Autodesk Fusion 360 part; units mm, degrees
note: some values were not read from the file. Set by a fixed rule: which sketch regions a step uses.
(part 2 of 4)
sketch "Sketch1 (2)" plane through (0, 0, 10) normal (0, 0, 1) x (-1, 0, 0)
  arc A0 (-15.295851, 2.795456) -> (-15.3295, 2.604619) centre (0, 0) ccw
  arc A1 (-16.525343, 1.694532) -> (-15.3295, 2.604619) centre (-16.413958, 2.788878) ccw
  line L0 (-16.525343, 1.694532) -> (-16.82626, 1.72516)
  spline S0 degree 3 poles (-19.988384, 0.681532) (-19.542306, 0.942193) (-19.068507, 1.175344) (-17.814234, 1.647532) (-17.303236, 1.701034) (-16.95637, 1.733314) (-16.879441, 1.730573) (-16.82626, 1.72516) knots -0.0362684 -0.0362684 -0.0362684 -0.0362684 -0.0284651 -0.0284651 -0.01603664 -0.01603664 0 0 0 0
  arc A2 (-19.988384, 0.681532) -> (-19.988384, -0.681532) centre (0, 0) ccw
  spline S1 degree 3 poles (-16.82626, -1.72516) (-17.047028, -1.747631) (-17.379442, -1.693217) (-17.83236, -1.598794) (-18.095918, -1.53109) (-18.963438, -1.226643) (-19.493456, -0.970738) (-19.988384, -0.681532) knots -0.3979886 -0.3979886 -0.3979886 -0.3979886 -0.27573533 -0.27573533 -0.17196952 -0.17196952 0 0 0 0
  line L1 (-16.82626, -1.72516) -> (-16.525343, -1.694532)
  arc A3 (-15.3295, -2.604619) -> (-16.525343, -1.694532) centre (-16.413958, -2.788878) ccw
  arc A4 (-15.3295, -2.604619) -> (-15.295851, -2.795456) centre (0, 0) ccw
  arc A5 (-16.108307, -4.059661) -> (-15.295851, -2.795456) centre (-16.377928, -2.993216) ccw
  line L2 (-16.108307, -4.059661) -> (-16.401552, -4.133799)
  spline S2 degree 3 poles (-19.016035, -6.196) (-18.68601, -5.79849) (-18.320527, -5.417351) (-17.303393, -4.544654) (-16.841511, -4.319606) (-16.526604, -4.170638) (-16.453377, -4.146902) (-16.401552, -4.133799) knots -0.0362684 -0.0362684 -0.0362684 -0.0362684 -0.0284651 -0.0284651 -0.01603664 -0.01603664 0 0 0 0
  arc A6 (-19.016035, -6.196) -> (-18.54984, -7.476861) centre (0, 0) ccw
  spline S3 degree 3 poles (-15.221473, -7.37604) (-15.421242, -7.472663) (-15.752219, -7.535223) (-16.210117, -7.601402) (-16.480937, -7.627923) (-17.400266, -7.638545) (-17.985845, -7.57935) (-18.54984, -7.476861) knots -0.3979886 -0.3979886 -0.3979886 -0.3979886 -0.27573533 -0.27573533 -0.17196952 -0.17196952 0 0 0 0
  line L3 (-15.221473, -7.37604) -> (-14.949179, -7.24434)
  arc A7 (-13.514186, -7.690539) -> (-14.949179, -7.24434) centre (-14.470223, -8.234593) ccw
  arc A8 (-13.514186, -7.690539) -> (-13.417296, -7.858359) centre (0, 0) ccw
  arc A9 (-13.748372, -9.324199) -> (-13.417296, -7.858359) centre (-14.366478, -8.414284) ccw
  line L4 (-13.748372, -9.324199) -> (-13.998575, -9.494162)
  spline S4 degree 3 poles (-15.750071, -12.326202) (-15.575905, -11.83979) (-15.36282, -11.356634) (-14.705508, -10.188687) (-14.348452, -9.819238) (-14.103485, -9.571549) (-14.042793, -9.524199) (-13.998575, -9.494162) knots -0.0362684 -0.0362684 -0.0362684 -0.0362684 -0.0284651 -0.0284651 -0.01603664 -0.01603664 0 0 0 0
  arc A10 (-15.750071, -12.326202) -> (-14.873911, -13.37037) centre (0, 0) ccw
  spline S5 degree 3 poles (-11.780751, -12.137261) (-11.935426, -12.296381) (-12.225046, -12.46837) (-12.632695, -12.687167) (-12.878111, -12.804715) (-13.738365, -13.129126) (-14.308875, -13.27378) (-14.873911, -13.37037) knots -0.3979886 -0.3979886 -0.3979886 -0.3979886 -0.27573533 -0.27573533 -0.17196952 -0.17196952 0 0 0 0
  line L5 (-11.780751, -12.137261) -> (-11.569923, -11.920373)
  arc A11 (-10.068861, -11.848867) -> (-11.569923, -11.920373) centre (-10.781165, -12.687094) ccw
  arc A12 (-10.068861, -11.848867) -> (-9.920417, -11.973427) centre (0, 0) ccw
  arc A13 (-9.73018, -13.464101) -> (-9.920417, -11.973427) centre (-10.622219, -12.820465) ccw
  line L6 (-9.73018, -13.464101) -> (-9.907163, -13.709388)
  spline S6 degree 3 poles (-10.584416, -16.969683) (-10.587116, -16.453037) (-10.552131, -15.92614) (-10.333921, -14.603813) (-10.124757, -14.134525) (-9.979279, -13.81799) (-9.938441, -13.752738) (-9.907163, -13.709388) knots -0.0362684 -0.0362684 -0.0362684 -0.0362684 -0.0284651 -0.0284651 -0.01603664 -0.01603664 0 0 0 0
  arc A14 (-10.584416, -16.969683) -> (-9.403968, -17.651215) centre (0, 0) ccw
  spline S7 degree 3 poles (-6.919097, -15.434549) (-7.010021, -15.636975) (-7.223352, -15.897647) (-7.531583, -16.242674) (-7.721996, -16.43707) (-8.419415, -17.03614) (-8.906044, -17.367197) (-9.403968, -17.651215) knots -0.3979886 -0.3979886 -0.3979886 -0.3979886 -0.27573533 -0.27573533 -0.17196952 -0.17196952 0 0 0 0
  line L7 (-6.919097, -15.434549) -> (-6.795164, -15.158633)
  arc A15 (-5.409084, -14.578046) -> (-6.795164, -15.158633) centre (-5.791739, -15.609344) ccw
  arc A16 (-5.409084, -14.578046) -> (-5.226989, -14.644323) centre (0, 0) ccw
  arc A17 (-4.538384, -15.980034) -> (-5.226989, -14.644323) centre (-5.596763, -15.680309) ccw
  line L8 (-4.538384, -15.980034) -> (-4.620801, -16.27106)
  spline S8 degree 3 poles (-4.142124, -19.566369) (-4.321365, -19.081804) (-4.468699, -18.574717) (-4.715911, -17.257505) (-4.679867, -16.74498) (-4.651423, -16.397778) (-4.635366, -16.322493) (-4.620801, -16.27106) knots -0.0362684 -0.0362684 -0.0362684 -0.0362684 -0.0284651 -0.0284651 -0.01603664 -0.01603664 0 0 0 0
  arc A18 (-4.142124, -19.566369) -> (-2.799769, -19.803063) centre (0, 0) ccw
  spline S9 degree 3 poles (-1.222898, -16.870202) (-1.239105, -17.091518) (-1.350415, -17.409433) (-1.522052, -17.839074) (-1.634494, -18.086871) (-2.084959, -18.888345) (-2.429013, -19.365873) (-2.799769, -19.803063) knots -0.3979886 -0.3979886 -0.3979886 -0.3979886 -0.27573533 -0.27573533 -0.17196952 -0.17196952 0 0 0 0
  line L9 (-1.222898, -16.870202) -> (-1.200807, -16.568538)
  arc A19 (-0.09689, -15.548898) -> (-1.200807, -16.568538) centre (-0.103745, -16.648877) ccw
  arc A20 (-0.09689, -15.548898) -> (0.09689, -15.548898) centre (0, 0) ccw
  arc A21 (1.200807, -16.568538) -> (0.09689, -15.548898) centre (0.103745, -16.648877) ccw
  line L10 (1.200807, -16.568538) -> (1.222898, -16.870202)
  spline S10 degree 3 poles (2.799769, -19.803063) (2.465607, -19.409025) (2.153724, -18.98291) (1.470907, -17.829687) (1.329484, -17.335743) (1.237462, -16.999751) (1.226802, -16.923515) (1.222898, -16.870202) knots -0.0362684 -0.0362684 -0.0362684 -0.0362684 -0.0284651 -0.0284651 -0.01603664 -0.01603664 0 0 0 0
  arc A22 (2.799769, -19.803063) -> (4.142124, -19.566369) centre (0, 0) ccw
  spline S11 degree 3 poles (4.620801, -16.27106) (4.681266, -16.484572) (4.685402, -16.821385) (4.671062, -17.283818) (4.650153, -17.555129) (4.500974, -18.462336) (4.340994, -19.02874) (4.142124, -19.566369) knots -0.3979886 -0.3979886 -0.3979886 -0.3979886 -0.27573533 -0.27573533 -0.17196952 -0.17196952 0 0 0 0
  line L11 (4.620801, -16.27106) -> (4.538384, -15.980034)
  arc A23 (5.226989, -14.644323) -> (4.538384, -15.980034) centre (5.596763, -15.680309) ccw
  arc A24 (5.226989, -14.644323) -> (5.409084, -14.578046) centre (0, 0) ccw
  arc A25 (6.795164, -15.158633) -> (5.409084, -14.578046) centre (5.791739, -15.609344) ccw
  line L12 (6.795164, -15.158633) -> (6.919097, -15.434549)
  spline S12 degree 3 poles (9.403968, -17.651215) (8.95519, -17.39523) (8.516376, -17.101484) (7.480313, -16.251345) (7.17848, -15.835559) (6.977091, -15.551304) (6.941, -15.483311) (6.919097, -15.434549) knots -0.0362684 -0.0362684 -0.0362684 -0.0362684 -0.0284651 -0.0284651 -0.01603664 -0.01603664 0 0 0 0
  arc A26 (9.403968, -17.651215) -> (10.584416, -16.969683) centre (0, 0) ccw
  spline S13 degree 3 poles (9.907163, -13.709388) (10.037006, -13.889344) (10.15609, -14.20443) (10.300776, -14.643879) (10.373922, -14.905979) (10.544023, -15.809497) (10.587412, -16.396459) (10.584416, -16.969683) knots -0.3979886 -0.3979886 -0.3979886 -0.3979886 -0.27573533 -0.27573533 -0.17196952 -0.17196952 0 0 0 0
  line L13 (9.907163, -13.709388) -> (9.73018, -13.464101)
  arc A27 (9.920417, -11.973427) -> (9.73018, -13.464101) centre (10.622219, -12.820465) ccw
  arc A28 (9.920417, -11.973427) -> (10.068861, -11.848867) centre (0, 0) ccw
  arc A29 (11.569923, -11.920373) -> (10.068861, -11.848867) centre (10.781165, -12.687094) ccw
  line L14 (11.569923, -11.920373) -> (11.780751, -12.137261)
  spline S14 degree 3 poles (14.873911, -13.37037) (14.364645, -13.283314) (13.851827, -13.157366) (12.587482, -12.712851) (12.161645, -12.425373) (11.87518, -12.22714) (11.818011, -12.175591) (11.780751, -12.137261) knots -0.0362684 -0.0362684 -0.0362684 -0.0362684 -0.0284651 -0.0284651 -0.01603664 -0.01603664 0 0 0 0
  arc A30 (14.873911, -13.37037) -> (15.750071, -12.326202) centre (0, 0) ccw
  spline S15 degree 3 poles (13.998575, -9.494162) (14.182136, -9.618856) (14.401804, -9.87421) (14.688065, -10.237672) (14.846443, -10.458949) (15.315307, -11.2498) (15.556832, -11.786523) (15.750071, -12.326202) knots -0.3979886 -0.3979886 -0.3979886 -0.3979886 -0.27573533 -0.27573533 -0.17196952 -0.17196952 0 0 0 0
  line L15 (13.998575, -9.494162) -> (13.748372, -9.324199)
  arc A31 (13.417296, -7.858359) -> (13.748372, -9.324199) centre (14.366478, -8.414284) ccw
  arc A32 (13.417296, -7.858359) -> (13.514186, -7.690539) centre (0, 0) ccw
  arc A33 (14.949179, -7.24434) -> (13.514186, -7.690539) centre (14.470223, -8.234593) ccw
  line L16 (14.949179, -7.24434) -> (15.221473, -7.37604)
  spline S16 degree 3 poles (18.54984, -7.476861) (18.041512, -7.569234) (17.516544, -7.626276) (16.176415, -7.641) (15.677936, -7.516504) (15.340947, -7.428202) (15.269595, -7.399316) (15.221473, -7.37604) knots -0.0362684 -0.0362684 -0.0362684 -0.0362684 -0.0284651 -0.0284651 -0.01603664 -0.01603664 0 0 0 0
  arc A34 (18.54984, -7.476861) -> (19.016035, -6.196) centre (0, 0) ccw
  spline S17 degree 3 poles (16.401552, -4.133799) (16.616691, -4.188191) (16.910448, -4.353016) (17.303757, -4.596651) (17.528264, -4.750414) (18.239339, -5.33321) (18.649869, -5.754959) (19.016035, -6.196) knots -0.3979886 -0.3979886 -0.3979886 -0.3979886 -0.27573533 -0.27573533 -0.17196952 -0.17196952 0 0 0 0
  line L17 (16.401552, -4.133799) -> (16.108307, -4.059661)
  arc A35 (15.295851, -2.795456) -> (16.108307, -4.059661) centre (16.377928, -2.993216) ccw
  arc A36 (15.295851, -2.795456) -> (15.3295, -2.604619) centre (0, 0) ccw
  arc A37 (16.525343, -1.694532) -> (15.3295, -2.604619) centre (16.413958, -2.788878) ccw
  line L18 (16.525343, -1.694532) -> (16.82626, -1.72516)
  spline S18 degree 3 poles (19.988384, -0.681532) (19.542306, -0.942193) (19.068507, -1.175344) (17.814234, -1.647532) (17.303236, -1.701034) (16.95637, -1.733314) (16.879441, -1.730573) (16.82626, -1.72516) knots -0.0362684 -0.0362684 -0.0362684 -0.0362684 -0.0284651 -0.0284651 -0.01603664 -0.01603664 0 0 0 0
  arc A38 (19.988384, -0.681532) -> (19.988384, 0.681532) centre (0, 0) ccw
  spline S19 degree 3 poles (16.82626, 1.72516) (17.047028, 1.747631) (17.379442, 1.693217) (17.83236, 1.598794) (18.095918, 1.53109) (18.963438, 1.226643) (19.493456, 0.970738) (19.988384, 0.681532) knots -0.3979886 -0.3979886 -0.3979886 -0.3979886 -0.27573533 -0.27573533 -0.17196952 -0.17196952 0 0 0 0
  line L19 (16.82626, 1.72516) -> (16.525343, 1.694532)
  arc A39 (15.3295, 2.604619) -> (16.525343, 1.694532) centre (16.413958, 2.788878) ccw
  arc A40 (15.3295, 2.604619) -> (15.295851, 2.795456) centre (0, 0) ccw
  arc A41 (16.108307, 4.059661) -> (15.295851, 2.795456) centre (16.377928, 2.993216) ccw
  line L20 (16.108307, 4.059661) -> (16.401552, 4.133799)
  spline S20 degree 3 poles (19.016035, 6.196) (18.68601, 5.79849) (18.320527, 5.417351) (17.303393, 4.544654) (16.841511, 4.319606) (16.526604, 4.170638) (16.453377, 4.146902) (16.401552, 4.133799) knots -0.0362684 -0.0362684 -0.0362684 -0.0362684 -0.0284651 -0.0284651 -0.01603664 -0.01603664 0 0 0 0
  arc A42 (19.016035, 6.196) -> (18.54984, 7.476861) centre (0, 0) ccw
  spline S21 degree 3 poles (15.221473, 7.37604) (15.421242, 7.472663) (15.752219, 7.535223) (16.210117, 7.601402) (16.480937, 7.627923) (17.400266, 7.638545) (17.985845, 7.57935) (18.54984, 7.476861) knots -0.3979886 -0.3979886 -0.3979886 -0.3979886 -0.27573533 -0.27573533 -0.17196952 -0.17196952 0 0 0 0
  line L21 (15.221473, 7.37604) -> (14.949179, 7.24434)
  arc A43 (13.514186, 7.690539) -> (14.949179, 7.24434) centre (14.470223, 8.234593) ccw
  arc A44 (13.514186, 7.690539) -> (13.417296, 7.858359) centre (0, 0) ccw
  arc A45 (13.748372, 9.324199) -> (13.417296, 7.858359) centre (14.366478, 8.414284) ccw
  line L22 (13.748372, 9.324199) -> (13.998575, 9.494162)
  spline S22 degree 3 poles (15.750071, 12.326202) (15.575905, 11.83979) (15.36282, 11.356634) (14.705508, 10.188687) (14.348452, 9.819238) (14.103485, 9.571549) (14.042793, 9.524199) (13.998575, 9.494162) knots -0.0362684 -0.0362684 -0.0362684 -0.0362684 -0.0284651 -0.0284651 -0.01603664 -0.01603664 0 0 0 0
  arc A46 (15.750071, 12.326202) -> (14.873911, 13.37037) centre (0, 0) ccw
  spline S23 degree 3 poles (11.780751, 12.137261) (11.935426, 12.296381) (12.225046, 12.46837) (12.632695, 12.687167) (12.878111, 12.804715) (13.738365, 13.129126) (14.308875, 13.27378) (14.873911, 13.37037) knots -0.3979886 -0.3979886 -0.3979886 -0.3979886 -0.27573533 -0.27573533 -0.17196952 -0.17196952 0 0 0 0
  line L23 (11.780751, 12.137261) -> (11.569923, 11.920373)
  arc A47 (10.068861, 11.848867) -> (11.569923, 11.920373) centre (10.781165, 12.687094) ccw
  arc A48 (10.068861, 11.848867) -> (9.920417, 11.973427) centre (0, 0) ccw
  arc A49 (9.73018, 13.464101) -> (9.920417, 11.973427) centre (10.622219, 12.820465) ccw
  line L24 (9.73018, 13.464101) -> (9.907163, 13.709388)
  spline S24 degree 3 poles (10.584416, 16.969683) (10.587116, 16.453037) (10.552131, 15.92614) (10.333921, 14.603813) (10.124757, 14.134525) (9.979279, 13.81799) (9.938441, 13.752738) (9.907163, 13.709388) knots -0.0362684 -0.0362684 -0.0362684 -0.0362684 -0.0284651 -0.0284651 -0.01603664 -0.01603664 0 0 0 0
  arc A50 (10.584416, 16.969683) -> (9.403968, 17.651215) centre (0, 0) ccw
  spline S25 degree 3 poles (6.919097, 15.434549) (7.010021, 15.636975) (7.223352, 15.897647) (7.531583, 16.242674) (7.721996, 16.43707) (8.419415, 17.03614) (8.906044, 17.367197) (9.403968, 17.651215) knots -0.3979886 -0.3979886 -0.3979886 -0.3979886 -0.27573533 -0.27573533 -0.17196952 -0.17196952 0 0 0 0
  line L25 (6.919097, 15.434549) -> (6.795164, 15.158633)
  arc A51 (5.409084, 14.578046) -> (6.795164, 15.158633) centre (5.791739, 15.609344) ccw
  arc A52 (5.409084, 14.578046) -> (5.226989, 14.644323) centre (0, 0) ccw
  arc A53 (4.538384, 15.980034) -> (5.226989, 14.644323) centre (5.596763, 15.680309) ccw
  line L26 (4.538384, 15.980034) -> (4.620801, 16.27106)
  spline S26 degree 3 poles (4.142124, 19.566369) (4.321365, 19.081804) (4.468699, 18.574717) (4.715911, 17.257505) (4.679867, 16.74498) (4.651423, 16.397778) (4.635366, 16.322493) (4.620801, 16.27106) knots -0.0362684 -0.0362684 -0.0362684 -0.0362684 -0.0284651 -0.0284651 -0.01603664 -0.01603664 0 0 0 0
  arc A54 (4.142124, 19.566369) -> (2.799769, 19.803063) centre (0, 0) ccw
  spline S27 degree 3 poles (1.222898, 16.870202) (1.239105, 17.091518) (1.350415, 17.409433) (1.522052, 17.839074) (1.634494, 18.086871) (2.084959, 18.888345) (2.429013, 19.365873) (2.799769, 19.803063) knots -0.3979886 -0.3979886 -0.3979886 -0.3979886 -0.27573533 -0.27573533 -0.17196952 -0.17196952 0 0 0 0
  line L27 (1.222898, 16.870202) -> (1.200807, 16.568538)
  arc A55 (0.09689, 15.548898) -> (1.200807, 16.568538) centre (0.103745, 16.648877) ccw
  arc A56 (0.09689, 15.548898) -> (-0.09689, 15.548898) centre (0, 0) ccw
  arc A57 (-1.200807, 16.568538) -> (-0.09689, 15.548898) centre (-0.103745, 16.648877) ccw
  line L28 (-1.200807, 16.568538) -> (-1.222898, 16.870202)
  spline S28 degree 3 poles (-2.799769, 19.803063) (-2.465607, 19.409025) (-2.153724, 18.98291) (-1.470907, 17.829687) (-1.329484, 17.335743) (-1.237462, 16.999751) (-1.226802, 16.923515) (-1.222898, 16.870202) knots -0.0362684 -0.0362684 -0.0362684 -0.0362684 -0.0284651 -0.0284651 -0.01603664 -0.01603664 0 0 0 0
  arc A58 (-2.799769, 19.803063) -> (-4.142124, 19.566369) centre (0, 0) ccw
  spline S29 degree 3 poles (-4.620801, 16.27106) (-4.681266, 16.484572) (-4.685402, 16.821385) (-4.671062, 17.283818) (-4.650153, 17.555129) (-4.500974, 18.462336) (-4.340994, 19.02874) (-4.142124, 19.566369) knots -0.3979886 -0.3979886 -0.3979886 -0.3979886 -0.27573533 -0.27573533 -0.17196952 -0.17196952 0 0 0 0
  line L29 (-4.620801, 16.27106) -> (-4.538384, 15.980034)
  arc A59 (-5.226989, 14.644323) -> (-4.538384, 15.980034) centre (-5.596763, 15.680309) ccw
  arc A60 (-5.226989, 14.644323) -> (-5.409084, 14.578046) centre (0, 0) ccw
  arc A61 (-6.795164, 15.158633) -> (-5.409084, 14.578046) centre (-5.791739, 15.609344) ccw
  line L30 (-6.795164, 15.158633) -> (-6.919097, 15.434549)
  spline S30 degree 3 poles (-9.403968, 17.651215) (-8.95519, 17.39523) (-8.516376, 17.101484) (-7.480313, 16.251345) (-7.17848, 15.835559) (-6.977091, 15.551304) (-6.941, 15.483311) (-6.919097, 15.434549) knots -0.0362684 -0.0362684 -0.0362684 -0.0362684 -0.0284651 -0.0284651 -0.01603664 -0.01603664 0 0 0 0
  arc A62 (-9.403968, 17.651215) -> (-10.584416, 16.969683) centre (0, 0) ccw
  spline S31 degree 3 poles (-9.907163, 13.709388) (-10.037006, 13.889344) (-10.15609, 14.20443) (-10.300776, 14.643879) (-10.373922, 14.905979) (-10.544023, 15.809497) (-10.587412, 16.396459) (-10.584416, 16.969683) knots -0.3979886 -0.3979886 -0.3979886 -0.3979886 -0.27573533 -0.27573533 -0.17196952 -0.17196952 0 0 0 0
  line L31 (-9.907163, 13.709388) -> (-9.73018, 13.464101)
  arc A63 (-9.920417, 11.973427) -> (-9.73018, 13.464101) centre (-10.622219, 12.820465) ccw
  arc A64 (-9.920417, 11.973427) -> (-10.068861, 11.848867) centre (0, 0) ccw
  arc A65 (-11.569923, 11.920373) -> (-10.068861, 11.848867) centre (-10.781165, 12.687094) ccw
  line L32 (-11.569923, 11.920373) -> (-11.780751, 12.137261)
  spline S32 degree 3 poles (-14.873911, 13.37037) (-14.364645, 13.283314) (-13.851827, 13.157366) (-12.587482, 12.712851) (-12.161645, 12.425373) (-11.87518, 12.22714) (-11.818011, 12.175591) (-11.780751, 12.137261) knots -0.0362684 -0.0362684 -0.0362684 -0.0362684 -0.0284651 -0.0284651 -0.01603664 -0.01603664 0 0 0 0
  arc A66 (-14.873911, 13.37037) -> (-15.750071, 12.326202) centre (0, 0) ccw
  spline S33 degree 3 poles (-13.998575, 9.494162) (-14.182136, 9.618856) (-14.401804, 9.87421) (-14.688065, 10.237672) (-14.846443, 10.458949) (-15.315307, 11.2498) (-15.556832, 11.786523) (-15.750071, 12.326202) knots -0.3979886 -0.3979886 -0.3979886 -0.3979886 -0.27573533 -0.27573533 -0.17196952 -0.17196952 0 0 0 0
  line L33 (-13.998575, 9.494162) -> (-13.748372, 9.324199)
  arc A67 (-13.417296, 7.858359) -> (-13.748372, 9.324199) centre (-14.366478, 8.414284) ccw
  arc A68 (-13.417296, 7.858359) -> (-13.514186, 7.690539) centre (0, 0) ccw
  arc A69 (-14.949179, 7.24434) -> (-13.514186, 7.690539) centre (-14.470223, 8.234593) ccw
  line L34 (-14.949179, 7.24434) -> (-15.221473, 7.37604)
  spline S34 degree 3 poles (-18.54984, 7.476861) (-18.041512, 7.569234) (-17.516544, 7.626276) (-16.176415, 7.641) (-15.677936, 7.516504) (-15.340947, 7.428202) (-15.269595, 7.399316) (-15.221473, 7.37604) knots -0.0362684 -0.0362684 -0.0362684 -0.0362684 -0.0284651 -0.0284651 -0.01603664 -0.01603664 0 0 0 0
  arc A70 (-18.54984, 7.476861) -> (-19.016035, 6.196) centre (0, 0) ccw
  spline S35 degree 3 poles (-16.401552, 4.133799) (-16.616691, 4.188191) (-16.910448, 4.353016) (-17.303757, 4.596651) (-17.528264, 4.750414) (-18.239339, 5.33321) (-18.649869, 5.754959) (-19.016035, 6.196) knots -0.3979886 -0.3979886 -0.3979886 -0.3979886 -0.27573533 -0.27573533 -0.17196952 -0.17196952 0 0 0 0
  line L35 (-16.401552, 4.133799) -> (-16.108307, 4.059661)
  arc A71 (-15.295851, 2.795456) -> (-16.108307, 4.059661) centre (-16.377928, 2.993216) ccw
  circle A72 centre (0, 0) radius 3.05
  dimension "d11" = 6.1
  constraint coincident A0.centre A2.centre
  measures "d11" diameter of A72
extrude "Extrude4" cut sketch "Sketch1 (2)" against normal blind 2 contours A72 picked at (-0.679049, -0.495194) in component "Spur Gear (18 teeth)"
move_face "OffsetFaces1" offset -0.1 1 faces at (0.679049, 0.495194, 8) in component "Spur Gear (18 teeth)"
sketch "Sketch2 (2)" plane through (0, 0, 10) normal (0, 0, 1) x (-1, 0, 0)
  circle A0 centre (0, 0) radius 3.05
  arc A1 (-15.295851, 2.795456) -> (-15.3295, 2.604619) centre (0, 0) ccw
  arc A2 (-16.525343, 1.694532) -> (-15.3295, 2.604619) centre (-16.413958, 2.788878) ccw
  line L0 (-16.525343, 1.694532) -> (-16.82626, 1.72516)
  spline S0 degree 3 poles (-19.988384, 0.681532) (-19.542306, 0.942193) (-19.068507, 1.175344) (-17.814234, 1.647532) (-17.303236, 1.701034) (-16.95637, 1.733314) (-16.879441, 1.730573) (-16.82626, 1.72516) knots -0.0362684 -0.0362684 -0.0362684 -0.0362684 -0.0284651 -0.0284651 -0.01603664 -0.01603664 0 0 0 0
  arc A3 (-19.988384, 0.681532) -> (-19.988384, -0.681532) centre (0, 0) ccw
  spline S1 degree 3 poles (-16.82626, -1.72516) (-17.047028, -1.747631) (-17.379442, -1.693217) (-17.83236, -1.598794) (-18.095918, -1.53109) (-18.963438, -1.226643) (-19.493456, -0.970738) (-19.988384, -0.681532) knots -0.3979886 -0.3979886 -0.3979886 -0.3979886 -0.27573533 -0.27573533 -0.17196952 -0.17196952 0 0 0 0
  line L1 (-16.82626, -1.72516) -> (-16.525343, -1.694532)
  arc A4 (-15.3295, -2.604619) -> (-16.525343, -1.694532) centre (-16.413958, -2.788878) ccw
  arc A5 (-15.3295, -2.604619) -> (-15.295851, -2.795456) centre (0, 0) ccw
  arc A6 (-16.108307, -4.059661) -> (-15.295851, -2.795456) centre (-16.377928, -2.993216) ccw
  line L2 (-16.108307, -4.059661) -> (-16.401552, -4.133799)
  spline S2 degree 3 poles (-19.016035, -6.196) (-18.68601, -5.79849) (-18.320527, -5.417351) (-17.303393, -4.544654) (-16.841511, -4.319606) (-16.526604, -4.170638) (-16.453377, -4.146902) (-16.401552, -4.133799) knots -0.0362684 -0.0362684 -0.0362684 -0.0362684 -0.0284651 -0.0284651 -0.01603664 -0.01603664 0 0 0 0
  arc A7 (-19.016035, -6.196) -> (-18.54984, -7.476861) centre (0, 0) ccw
  spline S3 degree 3 poles (-15.221473, -7.37604) (-15.421242, -7.472663) (-15.752219, -7.535223) (-16.210117, -7.601402) (-16.480937, -7.627923) (-17.400266, -7.638545) (-17.985845, -7.57935) (-18.54984, -7.476861) knots -0.3979886 -0.3979886 -0.3979886 -0.3979886 -0.27573533 -0.27573533 -0.17196952 -0.17196952 0 0 0 0
  line L3 (-15.221473, -7.37604) -> (-14.949179, -7.24434)
  arc A8 (-13.514186, -7.690539) -> (-14.949179, -7.24434) centre (-14.470223, -8.234593) ccw
  arc A9 (-13.514186, -7.690539) -> (-13.417296, -7.858359) centre (0, 0) ccw
  arc A10 (-13.748372, -9.324199) -> (-13.417296, -7.858359) centre (-14.366478, -8.414284) ccw
  line L4 (-13.748372, -9.324199) -> (-13.998575, -9.494162)
  spline S4 degree 3 poles (-15.750071, -12.326202) (-15.575905, -11.83979) (-15.36282, -11.356634) (-14.705508, -10.188687) (-14.348452, -9.819238) (-14.103485, -9.571549) (-14.042793, -9.524199) (-13.998575, -9.494162) knots -0.0362684 -0.0362684 -0.0362684 -0.0362684 -0.0284651 -0.0284651 -0.01603664 -0.01603664 0 0 0 0
  arc A11 (-15.750071, -12.326202) -> (-14.873911, -13.37037) centre (0, 0) ccw
  spline S5 degree 3 poles (-11.780751, -12.137261) (-11.935426, -12.296381) (-12.225046, -12.46837) (-12.632695, -12.687167) (-12.878111, -12.804715) (-13.738365, -13.129126) (-14.308875, -13.27378) (-14.873911, -13.37037) knots -0.3979886 -0.3979886 -0.3979886 -0.3979886 -0.27573533 -0.27573533 -0.17196952 -0.17196952 0 0 0 0
  line L5 (-11.780751, -12.137261) -> (-11.569923, -11.920373)
  arc A12 (-10.068861, -11.848867) -> (-11.569923, -11.920373) centre (-10.781165, -12.687094) ccw
  arc A13 (-10.068861, -11.848867) -> (-9.920417, -11.973427) centre (0, 0) ccw
  arc A14 (-9.73018, -13.464101) -> (-9.920417, -11.973427) centre (-10.622219, -12.820465) ccw
  line L6 (-9.73018, -13.464101) -> (-9.907163, -13.709388)
  spline S6 degree 3 poles (-10.584416, -16.969683) (-10.587116, -16.453037) (-10.552131, -15.92614) (-10.333921, -14.603813) (-10.124757, -14.134525) (-9.979279, -13.81799) (-9.938441, -13.752738) (-9.907163, -13.709388) knots -0.0362684 -0.0362684 -0.0362684 -0.0362684 -0.0284651 -0.0284651 -0.01603664 -0.01603664 0 0 0 0
  arc A15 (-10.584416, -16.969683) -> (-9.403968, -17.651215) centre (0, 0) ccw
  spline S7 degree 3 poles (-6.919097, -15.434549) (-7.010021, -15.636975) (-7.223352, -15.897647) (-7.531583, -16.242674) (-7.721996, -16.43707) (-8.419415, -17.03614) (-8.906044, -17.367197) (-9.403968, -17.651215) knots -0.3979886 -0.3979886 -0.3979886 -0.3979886 -0.27573533 -0.27573533 -0.17196952 -0.17196952 0 0 0 0
  line L7 (-6.919097, -15.434549) -> (-6.795164, -15.158633)
  arc A16 (-5.409084, -14.578046) -> (-6.795164, -15.158633) centre (-5.791739, -15.609344) ccw
  arc A17 (-5.409084, -14.578046) -> (-5.226989, -14.644323) centre (0, 0) ccw
  arc A18 (-4.538384, -15.980034) -> (-5.226989, -14.644323) centre (-5.596763, -15.680309) ccw
  line L8 (-4.538384, -15.980034) -> (-4.620801, -16.27106)
  spline S8 degree 3 poles (-4.142124, -19.566369) (-4.321365, -19.081804) (-4.468699, -18.574717) (-4.715911, -17.257505) (-4.679867, -16.74498) (-4.651423, -16.397778) (-4.635366, -16.322493) (-4.620801, -16.27106) knots -0.0362684 -0.0362684 -0.0362684 -0.0362684 -0.0284651 -0.0284651 -0.01603664 -0.01603664 0 0 0 0
  arc A19 (-4.142124, -19.566369) -> (-2.799769, -19.803063) centre (0, 0) ccw
  spline S9 degree 3 poles (-1.222898, -16.870202) (-1.239105, -17.091518) (-1.350415, -17.409433) (-1.522052, -17.839074) (-1.634494, -18.086871) (-2.084959, -18.888345) (-2.429013, -19.365873) (-2.799769, -19.803063) knots -0.3979886 -0.3979886 -0.3979886 -0.3979886 -0.27573533 -0.27573533 -0.17196952 -0.17196952 0 0 0 0
  line L9 (-1.222898, -16.870202) -> (-1.200807, -16.568538)
  arc A20 (-0.09689, -15.548898) -> (-1.200807, -16.568538) centre (-0.103745, -16.648877) ccw
  arc A21 (-0.09689, -15.548898) -> (0.09689, -15.548898) centre (0, 0) ccw
  arc A22 (1.200807, -16.568538) -> (0.09689, -15.548898) centre (0.103745, -16.648877) ccw
  line L10 (1.200807, -16.568538) -> (1.222898, -16.870202)
  spline S10 degree 3 poles (2.799769, -19.803063) (2.465607, -19.409025) (2.153724, -18.98291) (1.470907, -17.829687) (1.329484, -17.335743) (1.237462, -16.999751) (1.226802, -16.923515) (1.222898, -16.870202) knots -0.0362684 -0.0362684 -0.0362684 -0.0362684 -0.0284651 -0.0284651 -0.01603664 -0.01603664 0 0 0 0
  arc A23 (2.799769, -19.803063) -> (4.142124, -19.566369) centre (0, 0) ccw
  spline S11 degree 3 poles (4.620801, -16.27106) (4.681266, -16.484572) (4.685402, -16.821385) (4.671062, -17.283818) (4.650153, -17.555129) (4.500974, -18.462336) (4.340994, -19.02874) (4.142124, -19.566369) knots -0.3979886 -0.3979886 -0.3979886 -0.3979886 -0.27573533 -0.27573533 -0.17196952 -0.17196952 0 0 0 0
  line L11 (4.620801, -16.27106) -> (4.538384, -15.980034)
  arc A24 (5.226989, -14.644323) -> (4.538384, -15.980034) centre (5.596763, -15.680309) ccw
  arc A25 (5.226989, -14.644323) -> (5.409084, -14.578046) centre (0, 0) ccw
  arc A26 (6.795164, -15.158633) -> (5.409084, -14.578046) centre (5.791739, -15.609344) ccw
  line L12 (6.795164, -15.158633) -> (6.919097, -15.434549)
  spline S12 degree 3 poles (9.403968, -17.651215) (8.95519, -17.39523) (8.516376, -17.101484) (7.480313, -16.251345) (7.17848, -15.835559) (6.977091, -15.551304) (6.941, -15.483311) (6.919097, -15.434549) knots -0.0362684 -0.0362684 -0.0362684 -0.0362684 -0.0284651 -0.0284651 -0.01603664 -0.01603664 0 0 0 0
  arc A27 (9.403968, -17.651215) -> (10.584416, -16.969683) centre (0, 0) ccw
  spline S13 degree 3 poles (9.907163, -13.709388) (10.037006, -13.889344) (10.15609, -14.20443) (10.300776, -14.643879) (10.373922, -14.905979) (10.544023, -15.809497) (10.587412, -16.396459) (10.584416, -16.969683) knots -0.3979886 -0.3979886 -0.3979886 -0.3979886 -0.27573533 -0.27573533 -0.17196952 -0.17196952 0 0 0 0
  line L13 (9.907163, -13.709388) -> (9.73018, -13.464101)
  arc A28 (9.920417, -11.973427) -> (9.73018, -13.464101) centre (10.622219, -12.820465) ccw
  arc A29 (9.920417, -11.973427) -> (10.068861, -11.848867) centre (0, 0) ccw
  arc A30 (11.569923, -11.920373) -> (10.068861, -11.848867) centre (10.781165, -12.687094) ccw
  line L14 (11.569923, -11.920373) -> (11.780751, -12.137261)
  spline S14 degree 3 poles (14.873911, -13.37037) (14.364645, -13.283314) (13.851827, -13.157366) (12.587482, -12.712851) (12.161645, -12.425373) (11.87518, -12.22714) (11.818011, -12.175591) (11.780751, -12.137261) knots -0.0362684 -0.0362684 -0.0362684 -0.0362684 -0.0284651 -0.0284651 -0.01603664 -0.01603664 0 0 0 0
  arc A31 (14.873911, -13.37037) -> (15.750071, -12.326202) centre (0, 0) ccw
  spline S15 degree 3 poles (13.998575, -9.494162) (14.182136, -9.618856) (14.401804, -9.87421) (14.688065, -10.237672) (14.846443, -10.458949) (15.315307, -11.2498) (15.556832, -11.786523) (15.750071, -12.326202) knots -0.3979886 -0.3979886 -0.3979886 -0.3979886 -0.27573533 -0.27573533 -0.17196952 -0.17196952 0 0 0 0
  line L15 (13.998575, -9.494162) -> (13.748372, -9.324199)
  arc A32 (13.417296, -7.858359) -> (13.748372, -9.324199) centre (14.366478, -8.414284) ccw
  arc A33 (13.417296, -7.858359) -> (13.514186, -7.690539) centre (0, 0) ccw
  arc A34 (14.949179, -7.24434) -> (13.514186, -7.690539) centre (14.470223, -8.234593) ccw
  line L16 (14.949179, -7.24434) -> (15.221473, -7.37604)
  spline S16 degree 3 poles (18.54984, -7.476861) (18.041512, -7.569234) (17.516544, -7.626276) (16.176415, -7.641) (15.677936, -7.516504) (15.340947, -7.428202) (15.269595, -7.399316) (15.221473, -7.37604) knots -0.0362684 -0.0362684 -0.0362684 -0.0362684 -0.0284651 -0.0284651 -0.01603664 -0.01603664 0 0 0 0
  arc A35 (18.54984, -7.476861) -> (19.016035, -6.196) centre (0, 0) ccw
  spline S17 degree 3 poles (16.401552, -4.133799) (16.616691, -4.188191) (16.910448, -4.353016) (17.303757, -4.596651) (17.528264, -4.750414) (18.239339, -5.33321) (18.649869, -5.754959) (19.016035, -6.196) knots -0.3979886 -0.3979886 -0.3979886 -0.3979886 -0.27573533 -0.27573533 -0.17196952 -0.17196952 0 0 0 0
  line L17 (16.401552, -4.133799) -> (16.108307, -4.059661)
  arc A36 (15.295851, -2.795456) -> (16.108307, -4.059661) centre (16.377928, -2.993216) ccw
  arc A37 (15.295851, -2.795456) -> (15.3295, -2.604619) centre (0, 0) ccw
  arc A38 (16.525343, -1.694532) -> (15.3295, -2.604619) centre (16.413958, -2.788878) ccw
  line L18 (16.525343, -1.694532) -> (16.82626, -1.72516)
  spline S18 degree 3 poles (19.988384, -0.681532) (19.542306, -0.942193) (19.068507, -1.175344) (17.814234, -1.647532) (17.303236, -1.701034) (16.95637, -1.733314) (16.879441, -1.730573) (16.82626, -1.72516) knots -0.0362684 -0.0362684 -0.0362684 -0.0362684 -0.0284651 -0.0284651 -0.01603664 -0.01603664 0 0 0 0
  arc A39 (19.988384, -0.681532) -> (19.988384, 0.681532) centre (0, 0) ccw
  spline S19 degree 3 poles (16.82626, 1.72516) (17.047028, 1.747631) (17.379442, 1.693217) (17.83236, 1.598794) (18.095918, 1.53109) (18.963438, 1.226643) (19.493456, 0.970738) (19.988384, 0.681532) knots -0.3979886 -0.3979886 -0.3979886 -0.3979886 -0.27573533 -0.27573533 -0.17196952 -0.17196952 0 0 0 0
  line L19 (16.82626, 1.72516) -> (16.525343, 1.694532)
  arc A40 (15.3295, 2.604619) -> (16.525343, 1.694532) centre (16.413958, 2.788878) ccw
  arc A41 (15.3295, 2.604619) -> (15.295851, 2.795456) centre (0, 0) ccw
  arc A42 (16.108307, 4.059661) -> (15.295851, 2.795456) centre (16.377928, 2.993216) ccw
  line L20 (16.108307, 4.059661) -> (16.401552, 4.133799)
  spline S20 degree 3 poles (19.016035, 6.196) (18.68601, 5.79849) (18.320527, 5.417351) (17.303393, 4.544654) (16.841511, 4.319606) (16.526604, 4.170638) (16.453377, 4.146902) (16.401552, 4.133799) knots -0.0362684 -0.0362684 -0.0362684 -0.0362684 -0.0284651 -0.0284651 -0.01603664 -0.01603664 0 0 0 0
  arc A43 (19.016035, 6.196) -> (18.54984, 7.476861) centre (0, 0) ccw
  spline S21 degree 3 poles (15.221473, 7.37604) (15.421242, 7.472663) (15.752219, 7.535223) (16.210117, 7.601402) (16.480937, 7.627923) (17.400266, 7.638545) (17.985845, 7.57935) (18.54984, 7.476861) knots -0.3979886 -0.3979886 -0.3979886 -0.3979886 -0.27573533 -0.27573533 -0.17196952 -0.17196952 0 0 0 0
  line L21 (15.221473, 7.37604) -> (14.949179, 7.24434)
  arc A44 (13.514186, 7.690539) -> (14.949179, 7.24434) centre (14.470223, 8.234593) ccw
  arc A45 (13.514186, 7.690539) -> (13.417296, 7.858359) centre (0, 0) ccw
  arc A46 (13.748372, 9.324199) -> (13.417296, 7.858359) centre (14.366478, 8.414284) ccw
  line L22 (13.748372, 9.324199) -> (13.998575, 9.494162)
  spline S22 degree 3 poles (15.750071, 12.326202) (15.575905, 11.83979) (15.36282, 11.356634) (14.705508, 10.188687) (14.348452, 9.819238) (14.103485, 9.571549) (14.042793, 9.524199) (13.998575, 9.494162) knots -0.0362684 -0.0362684 -0.0362684 -0.0362684 -0.0284651 -0.0284651 -0.01603664 -0.01603664 0 0 0 0
  arc A47 (15.750071, 12.326202) -> (14.873911, 13.37037) centre (0, 0) ccw
  spline S23 degree 3 poles (11.780751, 12.137261) (11.935426, 12.296381) (12.225046, 12.46837) (12.632695, 12.687167) (12.878111, 12.804715) (13.738365, 13.129126) (14.308875, 13.27378) (14.873911, 13.37037) knots -0.3979886 -0.3979886 -0.3979886 -0.3979886 -0.27573533 -0.27573533 -0.17196952 -0.17196952 0 0 0 0
  line L23 (11.780751, 12.137261) -> (11.569923, 11.920373)
  arc A48 (10.068861, 11.848867) -> (11.569923, 11.920373) centre (10.781165, 12.687094) ccw
  arc A49 (10.068861, 11.848867) -> (9.920417, 11.973427) centre (0, 0) ccw
  arc A50 (9.73018, 13.464101) -> (9.920417, 11.973427) centre (10.622219, 12.820465) ccw
  line L24 (9.73018, 13.464101) -> (9.907163, 13.709388)
  spline S24 degree 3 poles (10.584416, 16.969683) (10.587116, 16.453037) (10.552131, 15.92614) (10.333921, 14.603813) (10.124757, 14.134525) (9.979279, 13.81799) (9.938441, 13.752738) (9.907163, 13.709388) knots -0.0362684 -0.0362684 -0.0362684 -0.0362684 -0.0284651 -0.0284651 -0.01603664 -0.01603664 0 0 0 0
  arc A51 (10.584416, 16.969683) -> (9.403968, 17.651215) centre (0, 0) ccw
  spline S25 degree 3 poles (6.919097, 15.434549) (7.010021, 15.636975) (7.223352, 15.897647) (7.531583, 16.242674) (7.721996, 16.43707) (8.419415, 17.03614) (8.906044, 17.367197) (9.403968, 17.651215) knots -0.3979886 -0.3979886 -0.3979886 -0.3979886 -0.27573533 -0.27573533 -0.17196952 -0.17196952 0 0 0 0
  line L25 (6.919097, 15.434549) -> (6.795164, 15.158633)
  arc A52 (5.409084, 14.578046) -> (6.795164, 15.158633) centre (5.791739, 15.609344) ccw
  arc A53 (5.409084, 14.578046) -> (5.226989, 14.644323) centre (0, 0) ccw
  arc A54 (4.538384, 15.980034) -> (5.226989, 14.644323) centre (5.596763, 15.680309) ccw
  line L26 (4.538384, 15.980034) -> (4.620801, 16.27106)
  spline S26 degree 3 poles (4.142124, 19.566369) (4.321365, 19.081804) (4.468699, 18.574717) (4.715911, 17.257505) (4.679867, 16.74498) (4.651423, 16.397778) (4.635366, 16.322493) (4.620801, 16.27106) knots -0.0362684 -0.0362684 -0.0362684 -0.0362684 -0.0284651 -0.0284651 -0.01603664 -0.01603664 0 0 0 0
  arc A55 (4.142124, 19.566369) -> (2.799769, 19.803063) centre (0, 0) ccw
  spline S27 degree 3 poles (1.222898, 16.870202) (1.239105, 17.091518) (1.350415, 17.409433) (1.522052, 17.839074) (1.634494, 18.086871) (2.084959, 18.888345) (2.429013, 19.365873) (2.799769, 19.803063) knots -0.3979886 -0.3979886 -0.3979886 -0.3979886 -0.27573533 -0.27573533 -0.17196952 -0.17196952 0 0 0 0
  line L27 (1.222898, 16.870202) -> (1.200807, 16.568538)
  arc A56 (0.09689, 15.548898) -> (1.200807, 16.568538) centre (0.103745, 16.648877) ccw
  arc A57 (0.09689, 15.548898) -> (-0.09689, 15.548898) centre (0, 0) ccw
  arc A58 (-1.200807, 16.568538) -> (-0.09689, 15.548898) centre (-0.103745, 16.648877) ccw
  line L28 (-1.200807, 16.568538) -> (-1.222898, 16.870202)
  spline S28 degree 3 poles (-2.799769, 19.803063) (-2.465607, 19.409025) (-2.153724, 18.98291) (-1.470907, 17.829687) (-1.329484, 17.335743) (-1.237462, 16.999751) (-1.226802, 16.923515) (-1.222898, 16.870202) knots -0.0362684 -0.0362684 -0.0362684 -0.0362684 -0.0284651 -0.0284651 -0.01603664 -0.01603664 0 0 0 0
  arc A59 (-2.799769, 19.803063) -> (-4.142124, 19.566369) centre (0, 0) ccw
  spline S29 degree 3 poles (-4.620801, 16.27106) (-4.681266, 16.484572) (-4.685402, 16.821385) (-4.671062, 17.283818) (-4.650153, 17.555129) (-4.500974, 18.462336) (-4.340994, 19.02874) (-4.142124, 19.566369) knots -0.3979886 -0.3979886 -0.3979886 -0.3979886 -0.27573533 -0.27573533 -0.17196952 -0.17196952 0 0 0 0
  line L29 (-4.620801, 16.27106) -> (-4.538384, 15.980034)
  arc A60 (-5.226989, 14.644323) -> (-4.538384, 15.980034) centre (-5.596763, 15.680309) ccw
  arc A61 (-5.226989, 14.644323) -> (-5.409084, 14.578046) centre (0, 0) ccw
  arc A62 (-6.795164, 15.158633) -> (-5.409084, 14.578046) centre (-5.791739, 15.609344) ccw
  line L30 (-6.795164, 15.158633) -> (-6.919097, 15.434549)
  spline S30 degree 3 poles (-9.403968, 17.651215) (-8.95519, 17.39523) (-8.516376, 17.101484) (-7.480313, 16.251345) (-7.17848, 15.835559) (-6.977091, 15.551304) (-6.941, 15.483311) (-6.919097, 15.434549) knots -0.0362684 -0.0362684 -0.0362684 -0.0362684 -0.0284651 -0.0284651 -0.01603664 -0.01603664 0 0 0 0
  arc A63 (-9.403968, 17.651215) -> (-10.584416, 16.969683) centre (0, 0) ccw
  spline S31 degree 3 poles (-9.907163, 13.709388) (-10.037006, 13.889344) (-10.15609, 14.20443) (-10.300776, 14.643879) (-10.373922, 14.905979) (-10.544023, 15.809497) (-10.587412, 16.396459) (-10.584416, 16.969683) knots -0.3979886 -0.3979886 -0.3979886 -0.3979886 -0.27573533 -0.27573533 -0.17196952 -0.17196952 0 0 0 0
  line L31 (-9.907163, 13.709388) -> (-9.73018, 13.464101)
  arc A64 (-9.920417, 11.973427) -> (-9.73018, 13.464101) centre (-10.622219, 12.820465) ccw
  arc A65 (-9.920417, 11.973427) -> (-10.068861, 11.848867) centre (0, 0) ccw
  arc A66 (-11.569923, 11.920373) -> (-10.068861, 11.848867) centre (-10.781165, 12.687094) ccw
  line L32 (-11.569923, 11.920373) -> (-11.780751, 12.137261)
  spline S32 degree 3 poles (-14.873911, 13.37037) (-14.364645, 13.283314) (-13.851827, 13.157366) (-12.587482, 12.712851) (-12.161645, 12.425373) (-11.87518, 12.22714) (-11.818011, 12.175591) (-11.780751, 12.137261) knots -0.0362684 -0.0362684 -0.0362684 -0.0362684 -0.0284651 -0.0284651 -0.01603664 -0.01603664 0 0 0 0
  arc A67 (-14.873911, 13.37037) -> (-15.750071, 12.326202) centre (0, 0) ccw
  spline S33 degree 3 poles (-13.998575, 9.494162) (-14.182136, 9.618856) (-14.401804, 9.87421) (-14.688065, 10.237672) (-14.846443, 10.458949) (-15.315307, 11.2498) (-15.556832, 11.786523) (-15.750071, 12.326202) knots -0.3979886 -0.3979886 -0.3979886 -0.3979886 -0.27573533 -0.27573533 -0.17196952 -0.17196952 0 0 0 0
  line L33 (-13.998575, 9.494162) -> (-13.748372, 9.324199)
  arc A68 (-13.417296, 7.858359) -> (-13.748372, 9.324199) centre (-14.366478, 8.414284) ccw
  arc A69 (-13.417296, 7.858359) -> (-13.514186, 7.690539) centre (0, 0) ccw
  arc A70 (-14.949179, 7.24434) -> (-13.514186, 7.690539) centre (-14.470223, 8.234593) ccw
  line L34 (-14.949179, 7.24434) -> (-15.221473, 7.37604)
  spline S34 degree 3 poles (-18.54984, 7.476861) (-18.041512, 7.569234) (-17.516544, 7.626276) (-16.176415, 7.641) (-15.677936, 7.516504) (-15.340947, 7.428202) (-15.269595, 7.399316) (-15.221473, 7.37604) knots -0.0362684 -0.0362684 -0.0362684 -0.0362684 -0.0284651 -0.0284651 -0.01603664 -0.01603664 0 0 0 0
  arc A71 (-18.54984, 7.476861) -> (-19.016035, 6.196) centre (0, 0) ccw
  spline S35 degree 3 poles (-16.401552, 4.133799) (-16.616691, 4.188191) (-16.910448, 4.353016) (-17.303757, 4.596651) (-17.528264, 4.750414) (-18.239339, 5.33321) (-18.649869, 5.754959) (-19.016035, 6.196) knots -0.3979886 -0.3979886 -0.3979886 -0.3979886 -0.27573533 -0.27573533 -0.17196952 -0.17196952 0 0 0 0
  line L35 (-16.401552, 4.133799) -> (-16.108307, 4.059661)
  arc A72 (-15.295851, 2.795456) -> (-16.108307, 4.059661) centre (-16.377928, 2.993216) ccw
  circle A73 centre (0, 0) radius 7
  dimension "d15" = 14
  constraint coincident A0.centre A1.centre
  measures "d15" diameter of A73
extrude "Extrude5" add sketch "Sketch2 (2)" along normal blind 9 contours A73 picked at (5.645917, -0.499292) in component "Spur Gear (18 teeth)"
sketch "Sketch3 (2)" plane through (0, 0, 0) normal (0, 1, 0) x (1, 0, 0)
  circle A0 centre (0, -14.5) radius 1.75
  dimension "d18" = 3.5
  measures "d18" diameter of A0
extrude "Extrude6" cut sketch "Sketch3 (2)" against normal blind 7 contours A0 picked at (0.525565, -14.420784) in component "Spur Gear (18 teeth)"
ref_plane "WorkPlane1" through (0, -6, 0) normal (0, 1, 0) x (0, 0, 1)
sketch "Sketch4" plane through (0, -6, 0) normal (0, 1, 0) x (1, 0, 0)
  line L0 (-7, -19) -> (7, -19)
  line L1 (7, -19) -> (7, -10)
  line L2 (7, -10) -> (-7, -10)
  line L3 (-7, -10) -> (-7, -19)
  dimension "d25" = 9
  dimension "d26" = 14
  constraint horizontal L0
  constraint vertical L1
  constraint horizontal L2
  constraint vertical L3
  measures "d25" distance of L0.end L1.end
  measures "d26" distance of L0.start L0.end
extrude "Extrude7" cut sketch "Sketch4" against normal blind 2.5 contours L0 L1 L2 L3 picked at (-2.333333, -13) in component "Spur Gear (18 teeth)"
move_face "OffsetFaces2" offset -0.2 1 faces at (-0.075976, -5.013824, 19) in component "Spur Gear (18 teeth)"
extrude "Extrude8" add 1 faces at (0.679049, 0.495194, 7.9) along direction (0, 0, 1) blind 2 in component "Spur Gear (18 teeth)"
extrude "Extrude9" add 1 faces at (0.043593, -6, 10.918298) along direction (0, -1, 0) blind 3.5 in component "Spur Gear (18 teeth)"
fillet "Fillet2" radius 0.5 1 edges at (2.843598, -1.102927, 18.8) in component "Spur Gear (18 teeth)"